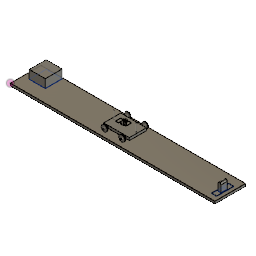
pendulo_CAD v3 (Autodesk Fusion 360 design; units mm, degrees)
Autodesk Fusion 360 part; units mm, degrees
note: some values were not read from the file. Chosen so that the rebuilt part matches the saved one: which face or edge a step refers to. Set by a fixed rule: which sketch regions a step uses.
sketch "base" plane through (0, 0, 0) normal (0, 1, 0) x (1, 0, 0)
  line L0 (0, 0) -> (1200, 0)
  line L1 (1200, 0) -> (1200, 180)
  line L2 (1200, 180) -> (0, 180)
  line L3 (0, 180) -> (0, 0)
  line L4 (1180, 30) -> (1150, 30)
  line L5 (1150, 30) -> (1150, 130)
  line L6 (1150, 130) -> (1180, 130)
  line L7 (1180, 130) -> (1180, 30)
  line L8 (1175, 60) -> (1158.2835, 60)
  line L9 (1158.2835, 60) -> (1158.2835, 96.8454)
  line L10 (1158.2835, 96.8454) -> (1175, 96.8454)
  line L11 (1175, 96.8454) -> (1175, 60)
  line L12 (35, 75) -> (130, 75)
  line L13 (130, 75) -> (130, 175)
  line L14 (130, 175) -> (35, 175)
  line L15 (35, 175) -> (35, 75)
  dimension "d1" = 180
  dimension "d2" = 1200
  dimension "d67" = 95
  measures "d2" distance of L0.start
extrude "Extrude22" add sketch "base" along normal blind 50 contours L12 L13 L14 L15 makes body 1
extrude "Extrude21" add sketch "base" along normal blind 50 separate body contours L8 L9 L10 L11 makes body 2
extrude "Extrude20" add sketch "base" along normal blind 1.5 separate body contours L4 L5 L6 L7 | L8 L9 L10 L11 makes body 3
sketch "carrinho" plane through (0, 0, 0) normal (0, 1, 0) x (1, 0, 0)
  line L0 (0, 0) -> (150, 0)
  line L1 (150, 0) -> (150, -100)
  line L2 (150, -100) -> (0, -100)
  line L3 (0, -100) -> (0, 0)
  circle A0 centre (140, -50) radius 1.5
  line L4 (82.5, -50) -> (64.5, -50)
  line L5 (64.5, -50) -> (64.5, -20)
  line L6 (64.5, -20) -> (82.5, -20)
  line L7 (82.5, -20) -> (82.5, -50)
  line L8 (64.5, -50) -> (82.5, -50)
  line L9 (82.5, -50) -> (82.5, -51.5)
  line L10 (82.5, -51.5) -> (64.5, -51.5)
  line L11 (64.5, -51.5) -> (64.5, -50)
  line L12 (75, -100) -> (75, 0)
  circle A1 centre (10, -50) radius 1.5
  dimension "d3" = 100
  dimension "d4" = 150
  dimension "d20" = 3
  dimension "d21" = 30
  dimension "d22" = 18
  dimension "d23" = 67.5
  dimension "d24" = 20
  dimension "d29" = 1.5
  dimension "d48" = 3
  measures "d20" diameter of A0
  measures "d48" diameter of A1
extrude "Extrude7" add sketch "carrinho" against normal blind 15 separate body contours L0 L2 L3 L5 L6 L10 L11 L12 | L0 L1 L2 L6 L7 L9 L10 L12 | L4 L5 L6 L8 L12 | L4 L6 L7 L8 L12 | L4 L8 L10 L11 L12 | L4 L8 L9 L10 L12 | A1 makes body 4
extrude "Extrude8" add sketch "carrinho" along normal blind 1.5 contours L4 L5 L6 L8 L12 | L4 L6 L7 L8 L12 bodies 4
extrude "Extrude9" add sketch "carrinho" along normal blind 30 contours L4 L8 L10 L11 L12 | L4 L8 L9 L10 L12 bodies 4
sketch "Sketch3" plane through (0, 0, 51.5) normal (0, 0, 1) x (1, 0, 0)
  line L0 (64.5, 0) -> (82.5, 0)
  line L1 (82.5, 0) -> (82.5, 30)
  line L2 (82.5, 30) -> (64.5, 30)
  line L3 (64.5, 30) -> (64.5, 0)
  circle A0 centre (73.3897, 20.1851) radius 2.75
  circle A1 centre (73.3897, 20.1851) radius 8.05
  dimension "d34" = 5.5
  dimension "d35" = 16.1
  measures "d34" diameter of A0
  measures "d35" diameter of A1
extrude "Extrude11" add sketch "Sketch3" along normal blind 19 contours A0 bodies 4
extrude "Extrude12" cut sketch "Sketch3" against normal blind 6 contours A0 bodies 4
extrude "Extrude13" add sketch "Sketch3" against normal blind 10 separate body contours A0 | A1 makes body 5
sketch "Sketch5" plane through (0, 0, 70.5) normal (0, 0, 1) x (1, 0, 0)
  circle A0 centre (73.3897, 20.1851) radius 2.75
  line L0 (82.5, 10.0824) -> (64.5, 10.0824)
  line L1 (64.5, 10.0824) -> (64.5, 40.0824)
  line L2 (64.5, 40.0824) -> (82.5, 40.0824)
  line L3 (82.5, 40.0824) -> (82.5, 10.0824)
  line L4 (82.5, 0) -> (82.5, 30)
  dimension "d42" = 30
  measures "d42" distance of origin
extrude "Extrude14" add sketch "Sketch5" along normal blind 1.5 separate body contours A0 | L0 L1 L2 L3 L4 makes body 6
sketch "Sketch6" plane through (82.5, 0, 0) normal (1, 0, 0) x (0, 0, -1)
  line L0 (-70.5, 10.0824) -> (-70.5, 40.0824)
  line L1 (-70.5, 40.0824) -> (-72, 40.0824)
  line L2 (-72, 40.0824) -> (-72, 10.0824)
  line L3 (-72, 10.0824) -> (-70.5, 10.0824)
  line L4 (-70.5, 40.0824) -> (-101, 40.0824)
  line L5 (-101, 40.0824) -> (-101, 38.5824)
  line L6 (-101, 38.5824) -> (-70.5, 38.5824)
  line L7 (-70.5, 38.5824) -> (-70.5, 40.0824)
  dimension "d45" = 1.5
extrude "Extrude15" add sketch "Sketch6" against normal blind 18 contours L2 L4 L5 L6 bodies 6
extrude "Extrude16" add sketch "carrinho" along normal blind 45 separate body contours A0 | A1 makes body 7 at (140.6169, 30, 48.6327) makes body 8 at (11.3173, 30, 49.2826)
move_body "Move1" bodies 4 7 6 8 5 to x (1, 0, 0) y (0, 1, 0) z (0, 0, 1) at (500, 35, -148)
extrude "Extrude17" add sketch "base" against normal blind 15 separate body contours L0 L1 L2 L3 | L4 L5 L6 L7 | L8 L9 L10 L11 | L12 L13 L14 L15 makes body 9
sketch "Sketch7" plane through (0, 0, -48) normal (0, 0, 1) x (1, 0, 0)
  line L0 (650, 35) -> (500, 35)
  line L1 (500, 35) -> (500, 20)
  line L2 (500, 20) -> (650, 20)
  line L3 (650, 20) -> (650, 35)
  circle A0 centre (625.6253, 28.4248) radius 5
  circle A1 centre (522.4288, 27.7322) radius 5
  dimension "d53" = 10
  dimension "d54" = 10
  measures "d53" diameter of A0
  measures "d54" diameter of A1
extrude "Extrude18" add sketch "Sketch7" along normal blind 25 separate body contours A0 | A1 makes body 10 at (624.7571, 33.3488, -31.3333) makes body 11 at (521.5606, 32.6562, -31.3333)
extrude "Extrude19" add 2 faces at (521.3897, 28.6964, -23) (624.5862, 29.389, -23) along direction (0, 0, -1) blind 150 on bodies 10 11 bodies 11 5 6 7 8 4 10
cylinder "CylinderPrimitive1" add diameter 35 height 5 placed x (1, 0, 0) y (0, 1, 0) z (0, 0, 1) at (625.6253, 28.4248, -23) separate body makes body 12
move_body "Move2" bodies 12 to x (1, 0, 0) y (0, 1, 0) z (0, 0, 1) at (0, 0, -10)
copy_body "CopyPasteBodies1" bodies 12 makes body 13
move_body "Move3" bodies 13 to x (1, 0, 0) y (0, 1, 0) z (0, 0, 1) at (-103, 0, 0)
copy_body "CopyPasteBodies2" bodies 12 13 makes body 14 makes body 15
move_body "Move4" bodies 14 15 to x (1, 0, 0) y (0, 1, 0) z (0, 0, 1) at (0, 0, -135)
move_body "Move5" bodies 8 14 13 5 7 12 11 6 15 to x (1, 0, 0) y (0, 1, 0) z (0, 0, 1) at (0, -10.8, 0)
move_body "Move6" bodies 6 to x (1, 0, 0) y (0, 1, 0) z (0, 0, 1) at (0, 0, -5)
copy_body "Body->Comp1" bodies 15 removing the originals makes body 16 in component "Component"
copy_body "Body->Comp2" bodies 8 removing the originals makes body 17 in component "Component'"
copy_body "Body->Comp3" bodies 13 removing the originals makes body 18 in component "Component''"
copy_body "Body->Comp4" bodies 14 removing the originals makes body 19 in component "Component'''"
copy_body "Body->Comp5" bodies 5 removing the originals makes body 20 in component "Component''''"
copy_body "Body->Comp6" bodies 11 removing the originals makes body 21 in component "Component'''''"
copy_body "Body->Comp7" bodies 12 removing the originals makes body 22 in component "Component''''''"
copy_body "Body->Comp8" bodies 7 removing the originals makes body 23 in component "Component'''''''"
copy_body "Body->Comp9" bodies 6 removing the originals makes body 24 in component "Component''''''''"
fillet "Fillet1" radius 10 1 edges at (1175, 50, -78.4227) on bodies 2
fillet "Fillet2" radius 7.5 1 edges at (1158.2835, 50, -78.4227) on bodies 2
component "Component" placed x (1, 0, 0) y (0, 1, 0) z (0, 0, 1) at (0, 0, 0)
component "Component'" placed x (1, 0, 0) y (0, 1, 0) z (0, 0, 1) at (0, 0, 0)
component "Component''" placed x (1, 0, 0) y (0, 1, 0) z (0, 0, 1) at (0, 0, 0)
component "Component'''" placed x (1, 0, 0) y (0, 1, 0) z (0, 0, 1) at (0, 0, 0)
component "Component''''" placed x (1, 0, 0) y (0, 1, 0) z (0, 0, 1) at (0, 0, 0)
component "Component'''''" placed x (1, 0, 0) y (0, 1, 0) z (0, 0, 1) at (0, 0, 0)
component "Component''''''" placed x (1, 0, 0) y (0, 1, 0) z (0, 0, 1) at (0, 0, 0)
component "Component'''''''" placed x (1, 0, 0) y (0, 1, 0) z (0, 0, 1) at (0, 0, 0)
component "Component''''''''" placed x (1, 0, 0) y (0, 1, 0) z (0, 0, 1) at (0, 0, 0)
named bodies: "carrinho"
